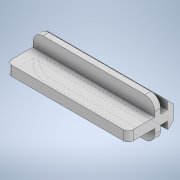
# Autodesk Inventor part: flag
Saved by Autodesk Inventor 2021 (Build 250183000, 183)
## iProperties
Created: 2025-06-24
Part Number: flag
Material: Generic
Document SubType Name: Modeling
Designer: Toby
Density: 1 g/cm^3
Appearance: Default
Author: Toby
Autodesk Inventor part; units mm, degrees
ref_plane "YZ Plane" through (0, 0, 0) normal (1, 0, 0) x (0, 1, 0)
ref_plane "XZ Plane" through (0, 0, 0) normal (0, 1, 0) x (-1, 0, 0)
ref_plane "XY Plane" through (0, 0, 0) normal (0, 0, 1) x (1, 0, 0)
sketch "Sketch1" plane through (0, 0, 0) normal (0, 0, 1) x (1, 0, 0)
  line L0 (-9.2369, 2.8715) -> (15.6631, 2.8715)
  line L1 (15.6631, 2.8715) -> (15.6631, -2.1285)
  line L2 (15.6631, -2.1285) -> (-9.2369, -2.1285)
  line L3 (-9.2369, -2.1285) -> (-9.2369, 2.8715)
  point P0 (0, 0)
  dimension "d0" = 24.9
  dimension "d1" = 5
  constraints: 8 end point, 2 parallel, 1 horizontal, 1 perpendicular
  measures "d0" distance of L0.start L0.end
  measures "d1" distance of L2.end L0.start
extrude "Extrusion1" add sketch "Sketch1" along normal blind 1.2
sketch "Sketch2" plane through (0, 0, 1.2) normal (0, 0, 1) x (1, 0, 0)
  line L0 (-9.2369, 2.8715) -> (-9.2369, -2.1285) projected
  line L1 (15.6631, -2.1285) -> (15.6631, 2.8715) projected
  line L2 (-9.2369, 1.3715) -> (15.6631, 1.3715)
  line L3 (15.6631, 1.3715) -> (15.6631, -0.6285)
  line L4 (15.6631, -0.6285) -> (-9.2369, -0.6285)
  line L5 (-9.2369, -0.6285) -> (-9.2369, 1.3715)
  line L6 (15.6631, 2.8715) -> (-9.2369, 2.8715) projected
  point P0 (0, 0)
  point P1 (15.6631, 1.3715)
  dimension "d4" = 2
  dimension "d5" = 1.5
  constraints: 8 end point, 2 parallel, 2 point on line, 1 horizontal, 1 perpendicular
  measures "d4" distance between parallel lines of L4 L2
  measures "d5" distance between parallel lines of L2 L6
extrude "Extrusion2" add sketch "Sketch2" along normal blind 8 contours L2 L1 L4 L0
chamfer "Chamfer1" distance 1 angle 45 2 edges at (3.2131, 2.8715, 0) (3.2131, -2.1285, 0)
fillet "Fillet4" radius 1 2 edges at (-9.2369, 0.3715, 9.2) (15.6631, 0.3715, 9.2)
sketch "Sketch3" plane through (-9.2369, 1.3715, 1.2) normal (0, 1, 0) x (1, 0, 0)
  line L0 (0, 0) -> (0, -7) projected
  line L1 (24.9, 0) -> (24.9, -7) projected
  line L2 (0, -1.4) -> (24.9, -1.4)
  line L3 (24.9, -1.4) -> (24.9, -2.6)
  line L4 (24.9, -2.6) -> (0, -2.6)
  line L5 (0, -2.6) -> (0, -1.4)
  line L6 (24.9, 0) -> (0, 0) projected
  point P0 (9.2369, 1.2)
  point P1 (0, -2.6)
  dimension "d15" = 1.4
  dimension "d16" = 1.2
  constraints: 8 end point, 2 parallel, 2 point on line, 1 horizontal, 1 perpendicular
  measures "d15" distance between parallel lines of L6 L2
  measures "d16" distance between parallel lines of L4 L2
extrude "Extrusion3" add sketch "Sketch3" along normal blind 3 contours L2 L1 L4 L0
sketch "Sketch4" plane through (-9.2369, -0.6285, 1.2) normal (0, -1, 0) x (1, 0, 0)
  line L0 (24.9, 2.6) -> (0, 2.6) projected
  line L1 (0, 1.4) -> (24.9, 1.4) projected
  line L2 (24.9, 2.6) -> (0, 2.6)
  line L3 (0, 2.6) -> (0, 1.4)
  line L4 (0, 1.4) -> (24.9, 1.4)
  line L5 (24.9, 1.4) -> (24.9, 2.6)
  point P0 (9.2369, -1.2)
  point P1 (0, 2.6)
  constraints: 8 end point, 2 parallel, 1 horizontal, 1 perpendicular
extrude "Extrusion4" add sketch "Sketch4" along normal blind 3
fillet "Fillet5" radius 2 4 edges at (-9.2369, 4.3715, 3.2) (-9.2369, -3.6285, 3.2) (15.6631, 4.3715, 3.2) (15.6631, -3.6285, 3.2)
body "Solid1"
